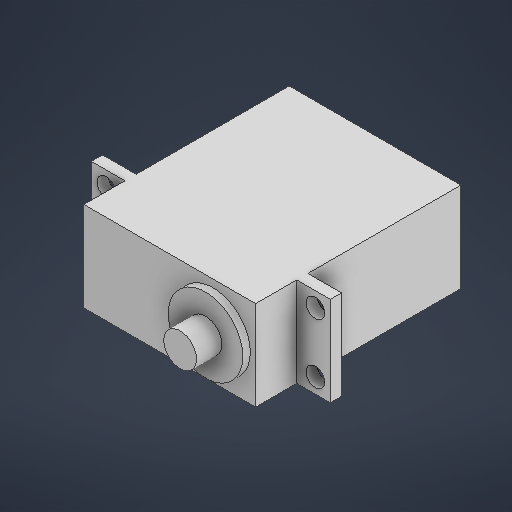
# Autodesk Inventor part: STS3032
Saved by Autodesk Inventor 2026 (Build 300175050, 175E)
## iProperties
Created: 2026-07-07
Part Number: STS3032
Material: 一般
Document SubType Name: Modeling
Designer: hanaj
Density: 1 g/cm^3
Appearance: 既定
Author: hanaj
Autodesk Inventor part; units mm, degrees
ref_plane "YZ Plane" through (0, 0, 0) normal (1, 0, 0) x (0, 1, 0)
ref_plane "XZ Plane" through (0, 0, 0) normal (0, 1, 0) x (-1, 0, 0)
ref_plane "XY Plane" through (0, 0, 0) normal (0, 0, 1) x (1, 0, 0)
sketch "スケッチ1" plane through (0, 0, 0) normal (0, 0, 1) x (1, 0, 0)
  line L0 (11.5, 6) -> (-11.5, 6)
  line L1 (-11.5, 6) -> (-11.5, -6)
  line L2 (-11.5, -6) -> (11.5, -6)
  line L3 (11.5, -6) -> (11.5, 6)
  line L4 (11.5, 6) -> (-11.5, -6) construction
  line L5 (-11.5, 6) -> (11.5, -6) construction
  point P0 (0, 0)
  dimension "d0" = 23
  dimension "d1" = 12
  constraints: 12 end point, 2 midpoint, 2 parallel, 1 horizontal, 1 perpendicular
  measures "d0" distance of L2.end L1.end
  measures "d1" distance of L1.end L0.end
extrude "押し出し1" add sketch "スケッチ1" along normal blind 20.5
sketch "スケッチ2" plane through (0, 0, 20.5) normal (0, 0, 1) x (1, 0, 0)
  line L0 (-16, 6) -> (16, 6)
  line L1 (16, 6) -> (16, -6)
  line L2 (16, -6) -> (-16, -6)
  line L3 (-16, -6) -> (-16, 6)
  line L4 (-16, 6) -> (16, -6) construction
  line L5 (16, 6) -> (-16, -6) construction
  point P0 (0, 0)
  dimension "d4" = 32
  dimension "d5" = 12
  constraints: 12 end point, 2 midpoint, 2 parallel, 1 horizontal, 1 perpendicular
  measures "d4" distance of L1.end L2.end
  measures "d5" distance of L0.end L1.end
extrude "押し出し2" add sketch "スケッチ2" along normal blind 1.5
sketch "スケッチ3" plane through (0, 0, 22) normal (0, 0, 1) x (1, 0, 0)
  line L0 (-11.5, 6) -> (-11.5, -6) projected
  line L1 (11.5, 6) -> (-11.5, 6) projected
  line L2 (11.5, -6) -> (11.5, 6) projected
  line L3 (-11.5, -6) -> (11.5, -6) projected
  point P0 (0, 0)
extrude "押し出し3" add sketch "スケッチ3" along normal blind 5.5
sketch "スケッチ4" plane through (0, 0, 27.5) normal (0, 0, 1) x (1, 0, 0)
  circle A0 centre (5.79, 0) radius 5
  line L0 (11.5, -6) -> (11.5, 6) projected
  line L1 (11.5, 6) -> (-11.5, 6) projected
  point P0 (0, 0)
  dimension "d10" = 5.71
  dimension "d11" = 6
  dimension "d12" = 10
  constraints: 1 centre point
  measures "d10" distance from line of L0 A0.centre
  measures "d11" distance from line of A0.centre L1
  measures "d12" diameter of A0
extrude "押し出し4" add sketch "スケッチ4" along normal blind 1
sketch "スケッチ5" plane through (5.79, 0, 28.5) normal (0, 0, 1) x (1, 0, 0)
  circle A0 centre (0, 0) radius 5 projected
  circle A1 centre (0, 0) radius 2.2
  point P0 (-5.79, 0)
  dimension "d15" = 4.4
  constraints: 1 centre point, 1 coincident
  measures "d15" diameter of A1
extrude "押し出し5" add sketch "スケッチ5" along normal blind 3.4 contours A1
sketch "スケッチ6" plane through (0, 0, 22) normal (0, 0, 1) x (1, 0, 0)
  line L0 (-19.7007, 0) -> (19.7007, 0)
  line L1 (0, -8.8838) -> (0, 8.8838)
  circle A0 centre (5.79, 0) radius 2.2 projected
  circle A1 centre (5.79, 0) radius 2.2 projected
  line L2 (-11.5, 6) -> (-16, 6) projected
  line L3 (16, 6) -> (11.5, 6) projected
  point P0 (0, 0)
  point P1 (-14, 4)
  point P2 (-14, -4)
  point P3 (14, 4)
  point P4 (14, -4)
  dimension "d18" = 19.79
  dimension "d19" = 2
  dimension "d20" = 8.21
  dimension "d21" = 2
  constraints: 4 end point, 2 midpoint, 2 symmetric about line, 1 horizontal, 1 vertical
  measures "d18" horizontal distance of point (-14, 4) A0.centre
  measures "d19" distance from line of L2 point (-14, 4)
  measures "d20" horizontal distance of point (14, 4) A0.centre
  measures "d21" distance from line of L3 point (14, 4)
hole "穴1" at (-14, 4, 22) at (-14, -4, 22) at (14, 4, 22) at (14, -4, 22) direction (0, 0, -1) diameter 2.5 end through all
